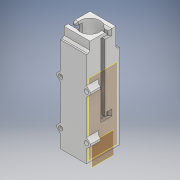
# Autodesk Inventor part: RescueKitThrow_pipe
Saved by Autodesk Inventor 2018.3 (Build 223284000, 284)
## iProperties
Created: 2019-02-10
Part Number: RescueKitThrow_pipe
Material: ABS プラスチック
Document SubType Name: Modeling
Designer: shun2
Density: 1.06 g/cm^3
Appearance: 滑らか - 白
Author: shun2
Autodesk Inventor part; units mm, degrees
ref_plane "YZ Plane" through (0, 0, 0) normal (1, 0, 0) x (0, 1, 0)
ref_plane "XZ Plane" through (0, 0, 0) normal (0, 1, 0) x (-1, 0, 0)
ref_plane "XY Plane" through (0, 0, 0) normal (0, 0, 1) x (1, 0, 0)
sketch "スケッチ1" plane through (0, 0, 0) normal (0, 0, 1) x (1, 0, 0)
  circle A0 centre (0, 0) radius 0.6
  line L0 (-0.6, 0) -> (0.6, 0)
  line L1 (-0.6, 0) -> (0.6, 0)
  line L2 (-13, 13) -> (13, 13)
  line L3 (13, 13) -> (13, -13)
  line L4 (13, -13) -> (-13, -13)
  line L5 (-13, -13) -> (-13, 13)
  dimension "d1" = 1.2
  dimension "d57" = 26
  dimension "d58" = 26
  constraints: 12 end point, 3 horizontal, 2 parallel, 2 point on circle, 1 centre point, 1 perpendicular
  measures "d1" diameter of A0
  measures "d57" distance of L3.end L4.end
  measures "d58" distance of L2.end L3.end
extrude "押し出し1" add sketch "スケッチ1" along normal blind 20
sketch "スケッチ2" plane through (0, 0, 20) normal (0, 0, 1) x (1, 0, 0)
  circle A0 centre (0, 0) radius 0.6 projected
  circle A1 centre (0, 0) radius 10
  line L0 (-0.6, 0) -> (0.6, 0)
  line L1 (13, 0) -> (13, 13)
  line L2 (-0.6, 0) -> (0.6, 0)
  line L3 (-13, 13) -> (13, 13)
  line L4 (13, 13) -> (13, -13)
  line L5 (13, -13) -> (-13, -13)
  line L6 (-13, -13) -> (-13, 13)
  dimension "d5" = 20
  dimension "d59" = 26
  dimension "d60" = 26
  constraints: 14 end point, 3 horizontal, 2 parallel, 2 perpendicular, 2 point on circle, 1 centre point, 1 coincident
  measures "d5" diameter of A1
  measures "d59" distance of L4.end L5.end
  measures "d60" distance of L3.end L4.end
extrude "押し出し2" add sketch "スケッチ2" along normal blind 80 contours L4 L5 L6 L3 L1
ref_plane "作業平面3" through (13, -13, 0) normal (1, 0, 0) x (0, 0, -1)
ref_plane "作業平面4" through (13, 0, 0) normal (1, 0, 0) x (0, 1, 0)
sketch "スケッチ3" plane through (13, 0, 0) normal (1, 0, 0) x (0, 1, 0)
  line L0 (-13, 0) -> (13, 0) projected
  line L1 (-13, 0) -> (-13, 65) projected
  line L2 (2, 94) -> (-2, 94)
  line L3 (-2, 94) -> (-2, 24)
  line L4 (-2, 24) -> (2, 24)
  line L5 (2, 24) -> (2, 94)
  line L6 (-13, 100) -> (13, 100) projected
  line L7 (13, 0) -> (13, 100) projected
  point P0 (0, 0)
  point P1 (0, 0)
  point P2 (0, 0)
  dimension "d80" = 4
  dimension "d81" = 70
  dimension "d90" = 6
  dimension "d131" = 11
  constraints: 8 end point, 2 parallel, 1 horizontal, 1 perpendicular, 1 other
  measures "d80" distance of L4.end L3.end
  measures "d81" distance of L3.end L2.end
  measures "d90" distance between parallel lines of L2 L6
  measures "d131" distance between parallel lines of L7 L5
extrude "押し出し3" cut sketch "スケッチ3" against normal blind 30
ref_plane "作業平面5" through (13, 0, 0) normal (1, 0, 0) x (0, 1, 0)
sketch "スケッチ4" plane through (13, 0, 0) normal (1, 0, 0) x (0, 1, 0)
  line L0 (-2, 94) -> (2, 94) projected
  line L1 (-2, 94) -> (7, 94)
  line L2 (7, 94) -> (7, 97)
  line L3 (4, 97) -> (-2, 97)
  line L4 (-2, 97) -> (-2, 94)
  line L5 (7, 94) -> (4, 94)
  line L6 (4, 97) -> (4, 100)
  line L7 (4, 100) -> (7, 100)
  line L8 (7, 100) -> (7, 94)
  line L9 (-2, 24) -> (-2, 94) projected
  line L10 (-2, 24) -> (7, 24)
  line L11 (7, 24) -> (7, 27)
  line L12 (4, 27) -> (-2, 27)
  line L13 (-2, 27) -> (-2, 24)
  line L14 (7, 24) -> (4, 24)
  line L15 (4, 27) -> (4, 30)
  line L16 (4, 30) -> (7, 30)
  line L17 (7, 30) -> (7, 24)
  point P0 (0, 0)
  point P1 (-1.25, 59)
  point P2 (-1.25, 10)
  dimension "d82" = 9
  dimension "d83" = 3
  dimension "d84" = 3
  dimension "d85" = 6
  dimension "d86" = 9
  dimension "d87" = 3
  dimension "d88" = 3
  dimension "d89" = 6
  constraints: 32 end point, 8 parallel, 4 horizontal, 4 perpendicular
  measures "d82" distance of L3.end L2.end
  measures "d83" distance of L2.end L1.end
  measures "d84" distance of L6.end L7.end
  measures "d85" distance of L5.end L6.end
  measures "d86" distance of L12.end L11.end
  measures "d87" distance of L11.end L10.end
  measures "d88" distance of L15.end L16.end
  measures "d89" distance of L14.end L15.end
extrude "押し出し4" cut sketch "スケッチ4" against normal blind 8
ref_plane "作業平面2" through (-13, 0, 0) normal (1, 0, 0) x (0, 1, 0)
sketch "スケッチ5" plane through (-13, 0, 0) normal (1, 0, 0) x (0, 1, 0)
  line L0 (6.25, 10) -> (-1.25, 10) projected
  line L1 (2, 94) -> (2, 27) projected
  line L2 (2, 94) -> (-7, 94)
  line L3 (-7, 94) -> (-7, 97)
  line L4 (-4, 97) -> (2, 97)
  line L5 (2, 97) -> (2, 94)
  line L6 (-7, 94) -> (-4, 94)
  line L7 (-4, 97) -> (-4, 100)
  line L8 (-4, 100) -> (-7, 100)
  line L9 (-7, 100) -> (-7, 94)
  line L10 (-2, 24) -> (2, 24) projected
  line L11 (2, 24) -> (-7, 24)
  line L12 (-7, 24) -> (-7, 27)
  line L13 (-4, 27) -> (2, 27)
  line L14 (2, 27) -> (2, 24)
  line L15 (-7, 24) -> (-4, 24)
  line L16 (-4, 27) -> (-4, 30)
  line L17 (-4, 30) -> (-7, 30)
  line L18 (-7, 30) -> (-7, 24)
  point P0 (0, 0)
  point P1 (1.25, 10)
  dimension "d91" = 9
  dimension "d92" = 3
  dimension "d93" = 3
  dimension "d94" = 6
  dimension "d95" = 9
  dimension "d96" = 3
  dimension "d97" = 3
  dimension "d98" = 6
  constraints: 32 end point, 8 parallel, 4 horizontal, 4 perpendicular, 1 point on line
  measures "d91" distance of L3.end L4.end
  measures "d92" distance of L2.end L3.end
  measures "d93" distance of L8.end L7.end
  measures "d94" distance of L7.end L6.end
  measures "d95" distance of L12.end L13.end
  measures "d96" distance of L11.end L12.end
  measures "d97" distance of L17.end L16.end
  measures "d98" distance of L16.end L15.end
extrude "押し出し5" cut sketch "スケッチ5" along normal blind 8
chamfer "面取り2" distance 2 angle 45 4 edges at (10.0707, 7, 100) (11.0826, 4, 100) (-11.0826, -4, 100) (-10.0707, -7, 100)
chamfer "面取り3" distance 2 angle 45 8 edges at (-13, -7, 96) (9.1652, 4, 97.5) (13, 7, 96) (-9.1652, -4, 97.5) (-13, -7, 27) (9.1652, 4, 28.5) (-9.1652, -4, 28.5) (13, 7, 27)
sketch "スケッチ6" plane through (0, 0, 20) normal (0, 0, 1) x (1, 0, 0)
  circle A0 centre (0, 0) radius 4.75
  circle A1 centre (0, 0) radius 0.6
  dimension "d65" = 9.5
  constraints: 2 centre point, 2 coincident
  measures "d65" diameter of A0
extrude "押し出し6" cut sketch "スケッチ6" against normal blind 15 contours A0 | A1
sketch "スケッチ7" plane through (-13, -13, 0) normal (0, -1, 0) x (1, 0, 0)
  line L0 (26, 0) -> (0, 0) projected
  line L1 (26, 0) -> (26, 100) projected
  line L2 (0, 100) -> (26, 100) projected
  line L3 (0, 0) -> (0, 100) projected
  line L4 (0, 0) -> (26, 0) projected
  line L5 (0, 0) -> (26, 0)
  line L6 (26, 0) -> (26, 90)
  line L7 (26, 90) -> (0, 90)
  line L8 (0, 90) -> (0, 0)
  point P0 (13, 0)
  dimension "d113" = 90
  constraints: 8 end point, 2 parallel, 1 horizontal, 1 perpendicular, 1 point on line
  measures "d113" distance of L6.end L5.end
extrude "押し出し7" add sketch "スケッチ7" along normal blind 3.5 contours L0 L3 L7 L1
sketch "スケッチ8" plane through (-13, -16.5, 0) normal (0, -1, 0) x (1, 0, 0)
  line L0 (-4, 16) -> (30, 16)
  line L1 (30, 16) -> (30, 10)
  line L2 (30, 10) -> (-4, 10)
  line L3 (-4, 10) -> (-4, 16)
  line L4 (0, 100) -> (0, 0) projected
  line L5 (0, 0) -> (26, 0) projected
  line L6 (-4, 61) -> (30, 61)
  line L7 (30, 61) -> (30, 55)
  line L8 (30, 55) -> (-4, 55)
  line L9 (-4, 55) -> (-4, 61)
  line L10 (0, 90) -> (0, 0) projected
  line L11 (26, 0) -> (26, 90) projected
  line L12 (0, 61) -> (26, 61)
  line L13 (26, 61) -> (26, 55)
  line L14 (26, 55) -> (0, 55)
  line L15 (0, 55) -> (0, 61)
  point P0 (13, 0)
  point P1 (0, 61)
  dimension "d101" = 34
  dimension "d102" = 6
  dimension "d107" = 4
  dimension "d110" = 10
  dimension "d126" = 34
  dimension "d127" = 6
  dimension "d128" = 55
  constraints: 24 end point, 6 parallel, 6 point on line, 3 horizontal, 3 perpendicular
  measures "d101" distance of L1.end L2.end
  measures "d102" distance of L0.end L1.end
  measures "d107" distance between parallel lines of L3 L4
  measures "d110" distance between parallel lines of L2 L5
  measures "d126" distance of L7.end L8.end
  measures "d127" distance of L6.end L7.end
  measures "d128" distance between parallel lines of L5 L8
extrude "押し出し8" add sketch "スケッチ8" against normal blind 10 contours L0 L4 L2 L3 | L0 L11 L2 L4 | L0 L1 L2 L11 | L8 L9 L6 L4 | L11 L6 L7 L8
sketch "スケッチ9" plane through (-13, -16.5, 0) normal (0, -1, 0) x (1, 0, 0)
  line L0 (26, 0) -> (26, 10) projected
  line L1 (30, 16) -> (30, 10) projected
  line L2 (-4, 10) -> (-4, 16) projected
  circle A0 centre (26, 13) radius 2.15
  circle A1 centre (0, 13) radius 2.15
  line L3 (0, 10) -> (0, 0) projected
  line L4 (26, 90) -> (0, 90) projected
  line L5 (26, 55) -> (30, 55) projected
  line L6 (30, 55) -> (30, 61) projected
  line L7 (30, 61) -> (26, 61) projected
  line L8 (-4, 61) -> (-4, 55) projected
  line L9 (-4, 55) -> (0, 55) projected
  line L10 (0, 0) -> (0, 100) projected
  circle A2 centre (0, 58) radius 2.15
  line L11 (26, 0) -> (26, 100) projected
  circle A3 centre (26, 58) radius 2.15
  line L12 (0, 61) -> (-4, 61) projected
  line L13 (0, 55) -> (0, 16) projected
  line L14 (0, 0) -> (26, 0) projected
  line L15 (26, 16) -> (26, 55) projected
  line L16 (30, 10) -> (26, 10) projected
  line L17 (26, 16) -> (30, 16) projected
  line L18 (26, 61) -> (26, 90) projected
  line L19 (0, 90) -> (0, 61) projected
  line L20 (-4, 16) -> (0, 16) projected
  line L21 (0, 10) -> (-4, 10) projected
  point P0 (13, 0)
  dimension "d105" = 4.3
  dimension "d106" = 4.3
  dimension "d129" = 4.3
  dimension "d130" = 4.3
  constraints: 4 centre point, 2 point on line
  measures "d105" diameter of A0
  measures "d106" diameter of A1
  measures "d129" diameter of A2
  measures "d130" diameter of A3
extrude "押し出し9" cut sketch "スケッチ9" against normal blind 8 contours L11 A0 | A0 L11 | L10 A1 | A1 L10 | A3 L11 | L11 A3 | A2 L10 | L10 A2
chamfer "面取り4" distance 2 angle 45 1 edges at (0, -13, 90)
chamfer "面取り5" distance 2 angle 45 20 edges at (-13, -11.5, 10) (13, -11.5, 10) (-13, -11.5, 16) (13, -11.5, 16) (-17, -11.5, 10) (17, -11.5, 10) (17, -11.5, 16) (-17, -11.5, 16) (-13, -6.5, 13) (13, -6.5, 13) (-17, -11.5, 55) (-17, -11.5, 61) (-13, -11.5, 55) (-13, -11.5, 61) (-13, -6.5, 58) (13, -11.5, 55) (17, -11.5, 55) (13, -11.5, 61) (13, -6.5, 58) (17, -11.5, 61)
sketch "スケッチ10" plane through (-13, 13, 0) normal (0, 1, 0) x (1, 0, 0)
  line L0 (0, 0) -> (26, 0) projected
  line L1 (0, 0) -> (26, 0)
  line L2 (26, 0) -> (26, -80)
  line L3 (26, -80) -> (0, -80)
  line L4 (0, -80) -> (0, 0)
  point P0 (13, 0)
  dimension "d120" = 80
  constraints: 8 end point, 2 parallel, 1 horizontal, 1 perpendicular
  measures "d120" distance of L1.end L2.end
extrude "押し出し10" add sketch "スケッチ10" along normal blind 3.5
chamfer "面取り6" distance 2 angle 45 1 edges at (0, 13, 80)
sketch "スケッチ11" plane through (0, 0, 20) normal (0, 0, 1) x (1, 0, 0)
  circle A0 centre (0, 0) radius 10
  dimension "d132" = 20
  constraints: 1 centre point, 1 coincident
  measures "d132" diameter of A0
extrude "押し出し11" cut sketch "スケッチ11" against normal blind 10
sketch "スケッチ12" plane through (-13, 0, 0) normal (1, 0, 0) x (0, 1, 0)
  point P0 (0, 0)
sketch "スケッチ13" plane through (0, 0, 0) normal (0, 0, -1) x (-1, 0, 0)
  circle A0 centre (0, 0) radius 0.6 projected
  circle A1 centre (0, 0) radius 0.6 projected
  line L0 (-13, 16.5) -> (-13, -16.5) projected
  line L1 (13, -16.5) -> (-13, -16.5) projected
  line L2 (13, -16.5) -> (13, 16.5) projected
  line L3 (-13, 16.5) -> (13, 16.5) projected
extrude "押し出し12" add sketch "スケッチ13" along normal blind 5
